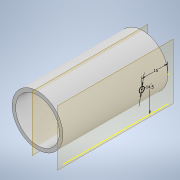
# Autodesk Inventor part: Peça1
Saved by Autodesk Inventor 2022 (Build 260153000, 153)
## iProperties
Created: 2023-10-22
Part Number: Peça1
Material: Genérico
Document SubType Name: Modeling
Designer: Daniel
Density: 1 g/cm^3
Appearance: Padrão
Author: Daniel
Autodesk Inventor part; units mm, degrees
ref_plane "XZ Plane" through (0, 0, 0) normal (0, 1, 0) x (-1, 0, 0)
ref_plane "XY Plane" through (0, 0, 0) normal (0, 0, 1) x (1, 0, 0)
sketch "Esboço1" plane through (0, 0, 0) normal (0, 0, 1) x (1, 0, 0)
  circle A0 centre (0, 0) radius 14.5
  dimension "d0" = 29
  constraints: 1 centre point, 1 coincident
  measures "d0" diameter of A0
extrude "Extrusão1" add sketch "Esboço1" along normal blind 2
sketch "Esboço2" plane through (0, 0, 2) normal (0, 0, 1) x (1, 0, 0)
  circle A0 centre (0, 0) radius 14.5 projected
  circle A1 centre (0, 0) radius 12.5
  dimension "d3" = 2
  constraints: 1 centre point
  measures "d3" radial gap between concentric circles of A0 A1
extrude "Extrusão2" add sketch "Esboço2" along normal blind 58
ref_plane "Plano de trabalho1" through (14.5, 0, 0) normal (1, 0, 0) x (0, 1, 0)
sketch "Esboço3" plane through (14.5, 0, 0) normal (1, 0, 0) x (0, 1, 0)
  circle A0 centre (0, 15) radius 1.5
  line L0 (-14.5, 0) -> (-14.5, 60) projected
  point P0 (0, 0)
  dimension "d7" = 3
  dimension "d8" = 15
  dimension "d9" = 14.5
  constraints: 1 centre point
  measures "d7" diameter of A0
  measures "d8" distance of point (0, 0) A0.centre
  measures "d9" distance from line of A0.centre L0
